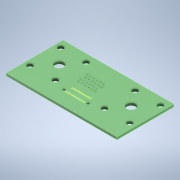
# Autodesk Inventor part: Cartridge PCB
Saved by Autodesk Inventor 2021 (Build 250183000, 183)
## iProperties
Created: 2020-04-22
Part Number: Cartridge PCB
Material: Generic
Document SubType Name: Modeling
Designer: jgray
Density: 1 g/cm^3
Appearance: Turquoise
Author: jgray
Autodesk Inventor part; units mm, degrees
ref_plane "YZ Plane" through (0, 0, 0) normal (1, 0, 0) x (0, 1, 0)
sketch "Sketch1" plane through (0, 0, 0) normal (0, 1, 0) x (-1, 0, 0)
  line L0 (-33.875, -17.375) -> (33.875, -17.375)
  line L1 (33.875, -17.375) -> (33.875, 17.375)
  line L2 (33.875, 17.375) -> (-33.875, 17.375)
  line L3 (-33.875, 17.375) -> (-33.875, -17.375)
  line L4 (-33.875, -17.375) -> (33.875, 17.375) construction
  line L5 (33.875, -17.375) -> (-33.875, 17.375) construction
  point P0 (0, 0)
  dimension "d0" = 67.75
  dimension "d1" = 34.75
  constraints: 12 end point, 2 midpoint, 2 parallel, 1 horizontal, 1 perpendicular
  measures "d0" distance of L2.end L1.end
  measures "d1" distance of L1.end L0.end
extrude "Extrusion1" add sketch "Sketch1" along normal blind 1.6
sketch "Sketch2" plane through (0, 1.6, 0) normal (0, 1, 0) x (1, 0, 0)
  line L0 (-33.875, 17.375) -> (-33.875, -17.375) projected
  line L1 (-33.875, -17.375) -> (33.875, -17.375) projected
  line L2 (33.875, -17.375) -> (33.875, 17.375) projected
  line L3 (33.875, 17.375) -> (-33.875, 17.375) projected
  line L4 (-35.405, 0) -> (38.2243, 0) construction
  line L5 (0, -28.3736) -> (0, 32.8828) construction
  line L6 (-37.7376, 3.2) -> (36.5002, 3.2) construction
  line L7 (22, -26.6494) -> (22, 29.2318) construction
  line L8 (-22, -24.9253) -> (-22, 32.8828) construction
  point P0 (0, 0)
  point P1 (-22, 3.2)
  point P2 (22, 3.2)
  dimension "d4" = 3.2
  dimension "d5" = 22
  dimension "d6" = 44
  constraints: 10 end point, 6 point on line, 3 vertical, 2 horizontal
  measures "d4" distance between parallel lines of L6 L4
  measures "d5" distance between parallel lines of L8 L5
  measures "d6" distance between parallel lines of L8 L7
hole "Hole1" at (-22, 1.6, -3.2) at (22, 1.6, -3.2) direction (0, -1, 0) diameter 5.5 end through all clearance for "Socket Head Cap Screw ISO 4762" size "M5" standard "ISO"
ref_plane "Work Plane1" through (0, 0, 17.375) normal (1, 0, 0) x (0, 0, -1)
ref_plane "Work Plane2" through (33.875, 0, 0) normal (0, 0, -1) x (-1, 0, 0)
sketch "Sketch3" plane through (0, 1.6, 0) normal (0, 1, 0) x (1, 0, 0)
  circle A0 centre (-22, 3.2) radius 2.75 projected
  circle A1 centre (22, 3.2) radius 2.75 projected
  line L0 (-33.875, 17.375) -> (-33.875, -17.375) projected
  line L1 (-33.875, -17.375) -> (33.875, -17.375) projected
  line L2 (33.875, -17.375) -> (33.875, 17.375) projected
  line L3 (33.875, 17.375) -> (-33.875, 17.375) projected
  line L4 (-39.0266, 3.2) -> (37.53, 3.2) construction
  line L5 (-15.4073, 6.3) -> (-2.3409, 6.3) construction
  line L6 (0, 20.8425) -> (0, -19.5249) construction
  line L7 (-36.2349, 0) -> (35.1135, 0) construction
  line L8 (-14.4073, 4.3) -> (-1.3409, 4.3) construction
  line L9 (-15.4073, 2.1) -> (-2.3409, 2.1) construction
  line L10 (-14.4073, 0.1) -> (-1.3409, 0.1) construction
  point P0 (0, 0)
  point P1 (-8, 6.3)
  point P2 (-6, 6.3)
  point P3 (-4, 6.3)
  point P4 (-2, 6.3)
  point P5 (0, 6.3)
  point P6 (2, 6.3)
  point P7 (-7, 4.3)
  point P8 (-5, 4.3)
  point P9 (-3, 4.3)
  point P10 (-1, 4.3)
  point P11 (1, 4.3)
  point P12 (3, 4.3)
  point P13 (-8, 2.1)
  point P14 (-6, 2.1)
  point P15 (-4, 2.1)
  point P16 (-2, 2.1)
  point P17 (0, 2.1)
  point P18 (2, 2.1)
  point P19 (-7, 0.1)
  point P20 (-5, 0.1)
  point P21 (-3, 0.1)
  point P22 (-1, 0.1)
  point P23 (1, 0.1)
  point P24 (3, 0.1)
  dimension "d16" = 2
  dimension "d25" = 2
  dimension "d35" = 2
  dimension "d49" = 2
  dimension "d51" = 1
  dimension "d52" = 2
  dimension "d53" = 1
  dimension "d54" = 2
  dimension "d55" = 2
  dimension "d56" = 2.2
  dimension "d57" = 8
  dimension "d111" = 1.1
  constraints: 14 end point, 9 horizontal, 7 point on line, 1 perpendicular, 1 vertical, 21 other
  measures "d16" distance of point (-8, 6.3) point (-6, 6.3)
  measures "d25" distance of point (-7, 4.3) point (-5, 4.3)
  measures "d35" distance of point (-8, 2.1) point (-6, 2.1)
  measures "d49" distance of point (-7, 0.1) point (-5, 0.1)
  measures "d51" horizontal distance of point (2, 6.3) point (3, 4.3)
  measures "d52" horizontal distance of point (-6, 6.3) point (-8, 2.1)
  measures "d53" horizontal distance of point (3, 0.1) point (2, 2.1)
  measures "d54" distance between parallel lines of L8 L5
  measures "d55" distance between parallel lines of L10 L9
  measures "d56" vertical distance of point (2, 2.1) point (3, 4.3)
  measures "d57" distance from line of point (-8, 6.3) L6
  measures "d111" distance from line of point (1, 4.3) L4
hole "Hole2" at (-8, 1.6, -6.3) at (-6, 1.6, -6.3) at (-4, 1.6, -6.3) at (-2, 1.6, -6.3) at (0, 1.6, -6.3) at (2, 1.6, -6.3) at (3, 1.6, -4.3) at (1, 1.6, -4.3) at (-1, 1.6, -4.3) at (-3, 1.6, -4.3) at (-5, 1.6, -4.3) at (-7, 1.6, -4.3) at (2, 1.6, -2.1) at (0, 1.6, -2.1) at (-2, 1.6, -2.1) at (-4, 1.6, -2.1) at (-6, 1.6, -2.1) at (-8, 1.6, -2.1) at (3, 1.6, -0.1) at (1, 1.6, -0.1) at (-1, 1.6, -0.1) at (-3, 1.6, -0.1) at (-5, 1.6, -0.1) at (-7, 1.6, -0.1) direction (0, -1, 0) diameter 0.8 end through all
sketch "Sketch4" plane through (0, 1.6, 0) normal (0, 1, 0) x (1, 0, 0)
  line L0 (0, 23.9201) -> (0, -23.9201) construction
  line L1 (-40.4387, 0) -> (47.2346, 0) construction
  line L2 (-12.2121, -8.55) -> (19.9504, -8.55) construction
  line L3 (-12.6831, -7.05) -> (19.9504, -7.05) construction
  line L4 (-42.6463, 3.2) -> (39.0543, 3.2) construction
  circle A0 centre (-5, 0.1) radius 0.4 construction
  circle A1 centre (-1, 0.1) radius 0.4 construction
  circle A2 centre (3, 0.1) radius 0.4 construction
  circle A3 centre (-6, 2.1) radius 0.4 construction
  circle A4 centre (-2, 2.1) radius 0.4 construction
  circle A5 centre (2, 2.1) radius 0.4 construction
  circle A6 centre (-5, 4.3) radius 0.4 construction
  circle A7 centre (-1, 4.3) radius 0.4 construction
  circle A8 centre (3, 4.3) radius 0.4 construction
  circle A9 centre (0, 6.3) radius 0.4 construction
  circle A10 centre (-4, 6.3) radius 0.4 construction
  circle A11 centre (-8, 6.3) radius 0.4 construction
  circle A12 centre (-6, 6.3) radius 0.4 construction
  circle A13 centre (-2, 6.3) radius 0.4 construction
  circle A14 centre (2, 6.3) radius 0.4 construction
  circle A15 centre (1, 4.3) radius 0.4 construction
  circle A16 centre (-3, 4.3) radius 0.4 construction
  circle A17 centre (-7, 4.3) radius 0.4 construction
  circle A18 centre (0, 2.1) radius 0.4 construction
  circle A19 centre (-4, 2.1) radius 0.4 construction
  circle A20 centre (-8, 2.1) radius 0.4 construction
  circle A21 centre (1, 0.1) radius 0.4 construction
  circle A22 centre (-3, 0.1) radius 0.4 construction
  circle A23 centre (-7, 0.1) radius 0.4 construction
  circle A24 centre (-22, 3.2) radius 2.75 construction
  circle A25 centre (22, 3.2) radius 2.75 construction
  line L5 (-33.875, 17.375) -> (-33.875, -17.375) construction
  line L6 (-33.875, -17.375) -> (33.875, -17.375) construction
  line L7 (33.875, -17.375) -> (33.875, 17.375) construction
  line L8 (33.875, 17.375) -> (-33.875, 17.375) construction
  point P0 (0, 0)
  point P1 (0, 0)
  point P2 (-7.4, -8.55)
  point P3 (7.4, -8.55)
  dimension "d65" = 1.5
  dimension "d66" = 14.8
  dimension "d67" = 10.25
  constraints: 10 end point, 6 point on line, 4 horizontal, 2 midpoint, 1 symmetric about line, 1 vertical
  measures "d65" distance between parallel lines of L3 L2
  measures "d66" distance of point (7.4, -8.55) point (-7.4, -8.55)
  measures "d67" distance between parallel lines of L4 L3
hole "Hole3" at (-7.4, 1.6, 8.55) at (7.4, 1.6, 8.55) direction (0, -1, 0) diameter 1.45 end through all
sketch "Sketch5" plane through (0, 1.6, 0) normal (0, 1, 0) x (1, 0, 0)
  line L0 (-11.5772, -5.15) -> (25.3732, -5.15) construction
  line L1 (-5.35, -5.7) -> (-5.85, -5.7)
  line L2 (-5.85, -5.7) -> (-5.85, -4.6)
  line L3 (-5.85, -4.6) -> (-5.35, -4.6)
  line L4 (-5.35, -4.6) -> (-5.35, -5.7)
  line L5 (-5.35, -5.7) -> (-5.85, -4.6) construction
  line L6 (-5.85, -5.7) -> (-5.35, -4.6) construction
  line L7 (0, 27.1403) -> (0, -35.4956) construction
  line L8 (-12.2121, -8.55) -> (19.9504, -8.55) construction
  line L9 (-12.6831, -7.05) -> (19.9504, -7.05) construction
  circle A0 centre (-7.4, -8.55) radius 0.725 construction
  circle A1 centre (7.4, -8.55) radius 0.725 construction
  circle A2 centre (-5, 0.1) radius 0.4 construction
  circle A3 centre (-1, 0.1) radius 0.4 construction
  circle A4 centre (3, 0.1) radius 0.4 construction
  circle A5 centre (-6, 2.1) radius 0.4 construction
  circle A6 centre (-2, 2.1) radius 0.4 construction
  circle A7 centre (2, 2.1) radius 0.4 construction
  circle A8 centre (-5, 4.3) radius 0.4 construction
  circle A9 centre (-1, 4.3) radius 0.4 construction
  circle A10 centre (3, 4.3) radius 0.4 construction
  circle A11 centre (0, 6.3) radius 0.4 construction
  circle A12 centre (-4, 6.3) radius 0.4 construction
  circle A13 centre (-8, 6.3) radius 0.4 construction
  circle A14 centre (-6, 6.3) radius 0.4 construction
  circle A15 centre (-2, 6.3) radius 0.4 construction
  circle A16 centre (2, 6.3) radius 0.4 construction
  circle A17 centre (1, 4.3) radius 0.4 construction
  circle A18 centre (-3, 4.3) radius 0.4 construction
  circle A19 centre (-7, 4.3) radius 0.4 construction
  circle A20 centre (0, 2.1) radius 0.4 construction
  circle A21 centre (-4, 2.1) radius 0.4 construction
  circle A22 centre (-8, 2.1) radius 0.4 construction
  circle A23 centre (1, 0.1) radius 0.4 construction
  circle A24 centre (-3, 0.1) radius 0.4 construction
  circle A25 centre (-7, 0.1) radius 0.4 construction
  circle A26 centre (-22, 3.2) radius 2.75 construction
  circle A27 centre (22, 3.2) radius 2.75 construction
  line L10 (-33.875, 17.375) -> (-33.875, -17.375) construction
  line L11 (-33.875, -17.375) -> (33.875, -17.375) construction
  line L12 (33.875, -17.375) -> (33.875, 17.375) construction
  line L13 (33.875, 17.375) -> (-33.875, 17.375) construction
  line L14 (-5.05, -5.7) -> (-5.05, -4.6)
  line L15 (-5.05, -4.6) -> (-4.55, -4.6)
  line L16 (-4.55, -5.7) -> (-5.05, -4.6) construction
  line L17 (-5.05, -5.7) -> (-4.55, -4.6) construction
  line L18 (-4.55, -4.6) -> (-4.55, -5.7)
  line L19 (-4.55, -5.7) -> (-5.05, -5.7)
  line L20 (-4.25, -5.7) -> (-4.25, -4.6)
  line L21 (-4.25, -4.6) -> (-3.75, -4.6)
  line L22 (-3.75, -5.7) -> (-4.25, -4.6) construction
  line L23 (-4.25, -5.7) -> (-3.75, -4.6) construction
  line L24 (-3.75, -4.6) -> (-3.75, -5.7)
  line L25 (-3.75, -5.7) -> (-4.25, -5.7)
  line L26 (-3.45, -5.7) -> (-3.45, -4.6)
  line L27 (-3.45, -4.6) -> (-2.95, -4.6)
  line L28 (-2.95, -5.7) -> (-3.45, -4.6) construction
  line L29 (-3.45, -5.7) -> (-2.95, -4.6) construction
  line L30 (-2.95, -4.6) -> (-2.95, -5.7)
  line L31 (-2.95, -5.7) -> (-3.45, -5.7)
  line L32 (-2.65, -5.7) -> (-2.65, -4.6)
  line L33 (-2.65, -4.6) -> (-2.15, -4.6)
  line L34 (-2.15, -5.7) -> (-2.65, -4.6) construction
  line L35 (-2.65, -5.7) -> (-2.15, -4.6) construction
  line L36 (-2.15, -4.6) -> (-2.15, -5.7)
  line L37 (-2.15, -5.7) -> (-2.65, -5.7)
  line L38 (-1.85, -5.7) -> (-1.85, -4.6)
  line L39 (-1.85, -4.6) -> (-1.35, -4.6)
  line L40 (-1.35, -5.7) -> (-1.85, -4.6) construction
  line L41 (-1.85, -5.7) -> (-1.35, -4.6) construction
  line L42 (-1.35, -4.6) -> (-1.35, -5.7)
  line L43 (-1.35, -5.7) -> (-1.85, -5.7)
  line L44 (-1.05, -5.7) -> (-1.05, -4.6)
  line L45 (-1.05, -4.6) -> (-0.55, -4.6)
  line L46 (-0.55, -5.7) -> (-1.05, -4.6) construction
  line L47 (-1.05, -5.7) -> (-0.55, -4.6) construction
  line L48 (-0.55, -4.6) -> (-0.55, -5.7)
  line L49 (-0.55, -5.7) -> (-1.05, -5.7)
  line L50 (-0.25, -5.7) -> (-0.25, -4.6)
  line L51 (-0.25, -4.6) -> (0.25, -4.6)
  line L52 (0.25, -5.7) -> (-0.25, -4.6) construction
  line L53 (-0.25, -5.7) -> (0.25, -4.6) construction
  line L54 (0.25, -4.6) -> (0.25, -5.7)
  line L55 (0.25, -5.7) -> (-0.25, -5.7)
  line L56 (0.55, -5.7) -> (0.55, -4.6)
  line L57 (0.55, -4.6) -> (1.05, -4.6)
  line L58 (1.05, -5.7) -> (0.55, -4.6) construction
  line L59 (0.55, -5.7) -> (1.05, -4.6) construction
  line L60 (1.05, -4.6) -> (1.05, -5.7)
  line L61 (1.05, -5.7) -> (0.55, -5.7)
  line L62 (1.35, -5.7) -> (1.35, -4.6)
  line L63 (1.35, -4.6) -> (1.85, -4.6)
  line L64 (1.85, -5.7) -> (1.35, -4.6) construction
  line L65 (1.35, -5.7) -> (1.85, -4.6) construction
  line L66 (1.85, -4.6) -> (1.85, -5.7)
  line L67 (1.85, -5.7) -> (1.35, -5.7)
  line L68 (2.15, -5.7) -> (2.15, -4.6)
  line L69 (2.15, -4.6) -> (2.65, -4.6)
  line L70 (2.65, -5.7) -> (2.15, -4.6) construction
  line L71 (2.15, -5.7) -> (2.65, -4.6) construction
  line L72 (2.65, -4.6) -> (2.65, -5.7)
  line L73 (2.65, -5.7) -> (2.15, -5.7)
  line L74 (2.95, -5.7) -> (2.95, -4.6)
  line L75 (2.95, -4.6) -> (3.45, -4.6)
  line L76 (3.45, -5.7) -> (2.95, -4.6) construction
  line L77 (2.95, -5.7) -> (3.45, -4.6) construction
  line L78 (3.45, -4.6) -> (3.45, -5.7)
  line L79 (3.45, -5.7) -> (2.95, -5.7)
  line L80 (3.75, -5.7) -> (3.75, -4.6)
  line L81 (3.75, -4.6) -> (4.25, -4.6)
  line L82 (4.25, -5.7) -> (3.75, -4.6) construction
  line L83 (3.75, -5.7) -> (4.25, -4.6) construction
  line L84 (4.25, -4.6) -> (4.25, -5.7)
  line L85 (4.25, -5.7) -> (3.75, -5.7)
  line L86 (4.55, -5.7) -> (4.55, -4.6)
  line L87 (4.55, -4.6) -> (5.05, -4.6)
  line L88 (5.05, -5.7) -> (4.55, -4.6) construction
  line L89 (4.55, -5.7) -> (5.05, -4.6) construction
  line L90 (5.05, -4.6) -> (5.05, -5.7)
  line L91 (5.05, -5.7) -> (4.55, -5.7)
  line L92 (5.35, -5.7) -> (5.35, -4.6)
  line L93 (5.35, -4.6) -> (5.85, -4.6)
  line L94 (5.85, -5.7) -> (5.35, -4.6) construction
  line L95 (5.35, -5.7) -> (5.85, -4.6) construction
  line L96 (5.85, -4.6) -> (5.85, -5.7)
  line L97 (5.85, -5.7) -> (5.35, -5.7)
  line L98 (-5.85, -9.5) -> (-5.85, -8.4)
  line L99 (-5.85, -8.4) -> (-5.35, -8.4)
  line L100 (-5.35, -9.5) -> (-5.85, -8.4) construction
  line L101 (-5.85, -9.5) -> (-5.35, -8.4) construction
  line L102 (-5.35, -8.4) -> (-5.35, -9.5)
  line L103 (-5.35, -9.5) -> (-5.85, -9.5)
  line L104 (-5.05, -9.5) -> (-5.05, -8.4)
  line L105 (-5.05, -8.4) -> (-4.55, -8.4)
  line L106 (-4.55, -9.5) -> (-5.05, -8.4) construction
  line L107 (-5.05, -9.5) -> (-4.55, -8.4) construction
  line L108 (-4.55, -8.4) -> (-4.55, -9.5)
  line L109 (-4.55, -9.5) -> (-5.05, -9.5)
  line L110 (-4.25, -9.5) -> (-4.25, -8.4)
  line L111 (-4.25, -8.4) -> (-3.75, -8.4)
  line L112 (-3.75, -9.5) -> (-4.25, -8.4) construction
  line L113 (-4.25, -9.5) -> (-3.75, -8.4) construction
  line L114 (-3.75, -8.4) -> (-3.75, -9.5)
  line L115 (-3.75, -9.5) -> (-4.25, -9.5)
  line L116 (-3.45, -9.5) -> (-3.45, -8.4)
  line L117 (-3.45, -8.4) -> (-2.95, -8.4)
  line L118 (-2.95, -9.5) -> (-3.45, -8.4) construction
  line L119 (-3.45, -9.5) -> (-2.95, -8.4) construction
  line L120 (-2.95, -8.4) -> (-2.95, -9.5)
  line L121 (-2.95, -9.5) -> (-3.45, -9.5)
  line L122 (-2.65, -9.5) -> (-2.65, -8.4)
  line L123 (-2.65, -8.4) -> (-2.15, -8.4)
  line L124 (-2.15, -9.5) -> (-2.65, -8.4) construction
  line L125 (-2.65, -9.5) -> (-2.15, -8.4) construction
  line L126 (-2.15, -8.4) -> (-2.15, -9.5)
  line L127 (-2.15, -9.5) -> (-2.65, -9.5)
  line L128 (-1.85, -9.5) -> (-1.85, -8.4)
  line L129 (-1.85, -8.4) -> (-1.35, -8.4)
  line L130 (-1.35, -9.5) -> (-1.85, -8.4) construction
  line L131 (-1.85, -9.5) -> (-1.35, -8.4) construction
  line L132 (-1.35, -8.4) -> (-1.35, -9.5)
  line L133 (-1.35, -9.5) -> (-1.85, -9.5)
  line L134 (-1.05, -9.5) -> (-1.05, -8.4)
  line L135 (-1.05, -8.4) -> (-0.55, -8.4)
  line L136 (-0.55, -9.5) -> (-1.05, -8.4) construction
  line L137 (-1.05, -9.5) -> (-0.55, -8.4) construction
  line L138 (-0.55, -8.4) -> (-0.55, -9.5)
  line L139 (-0.55, -9.5) -> (-1.05, -9.5)
  line L140 (-0.25, -9.5) -> (-0.25, -8.4)
  line L141 (-0.25, -8.4) -> (0.25, -8.4)
  line L142 (0.25, -9.5) -> (-0.25, -8.4) construction
  line L143 (-0.25, -9.5) -> (0.25, -8.4) construction
  line L144 (0.25, -8.4) -> (0.25, -9.5)
  line L145 (0.25, -9.5) -> (-0.25, -9.5)
  line L146 (0.55, -9.5) -> (0.55, -8.4)
  line L147 (0.55, -8.4) -> (1.05, -8.4)
  line L148 (1.05, -9.5) -> (0.55, -8.4) construction
  line L149 (0.55, -9.5) -> (1.05, -8.4) construction
  line L150 (1.05, -8.4) -> (1.05, -9.5)
  line L151 (1.05, -9.5) -> (0.55, -9.5)
  line L152 (1.35, -9.5) -> (1.35, -8.4)
  line L153 (1.35, -8.4) -> (1.85, -8.4)
  line L154 (1.85, -9.5) -> (1.35, -8.4) construction
  line L155 (1.35, -9.5) -> (1.85, -8.4) construction
  line L156 (1.85, -8.4) -> (1.85, -9.5)
  line L157 (1.85, -9.5) -> (1.35, -9.5)
  line L158 (2.15, -9.5) -> (2.15, -8.4)
  line L159 (2.15, -8.4) -> (2.65, -8.4)
  line L160 (2.65, -9.5) -> (2.15, -8.4) construction
  line L161 (2.15, -9.5) -> (2.65, -8.4) construction
  line L162 (2.65, -8.4) -> (2.65, -9.5)
  line L163 (2.65, -9.5) -> (2.15, -9.5)
  line L164 (2.95, -9.5) -> (2.95, -8.4)
  line L165 (2.95, -8.4) -> (3.45, -8.4)
  line L166 (3.45, -9.5) -> (2.95, -8.4) construction
  line L167 (2.95, -9.5) -> (3.45, -8.4) construction
  line L168 (3.45, -8.4) -> (3.45, -9.5)
  line L169 (3.45, -9.5) -> (2.95, -9.5)
  line L170 (3.75, -9.5) -> (3.75, -8.4)
  line L171 (3.75, -8.4) -> (4.25, -8.4)
  line L172 (4.25, -9.5) -> (3.75, -8.4) construction
  line L173 (3.75, -9.5) -> (4.25, -8.4) construction
  line L174 (4.25, -8.4) -> (4.25, -9.5)
  line L175 (4.25, -9.5) -> (3.75, -9.5)
  line L176 (4.55, -9.5) -> (4.55, -8.4)
  line L177 (4.55, -8.4) -> (5.05, -8.4)
  line L178 (5.05, -9.5) -> (4.55, -8.4) construction
  line L179 (4.55, -9.5) -> (5.05, -8.4) construction
  line L180 (5.05, -8.4) -> (5.05, -9.5)
  line L181 (5.05, -9.5) -> (4.55, -9.5)
  line L182 (5.35, -9.5) -> (5.35, -8.4)
  line L183 (5.35, -8.4) -> (5.85, -8.4)
  line L184 (5.85, -9.5) -> (5.35, -8.4) construction
  line L185 (5.35, -9.5) -> (5.85, -8.4) construction
  line L186 (5.85, -8.4) -> (5.85, -9.5)
  line L187 (5.85, -9.5) -> (5.35, -9.5)
  point P0 (0, 0)
  point P1 (-5.6, -5.15)
  point P2 (-4.8, -5.15)
  point P3 (-4, -5.15)
  point P4 (-3.2, -5.15)
  point P5 (-2.4, -5.15)
  point P6 (-1.6, -5.15)
  point P7 (-0.8, -5.15)
  point P8 (0, -5.15)
  point P9 (0.8, -5.15)
  point P10 (1.6, -5.15)
  point P11 (2.4, -5.15)
  point P12 (3.2, -5.15)
  point P13 (4, -5.15)
  point P14 (4.8, -5.15)
  point P15 (5.6, -5.15)
  point P16 (-5.6, -8.95)
  point P17 (-4.8, -8.95)
  point P18 (-4, -8.95)
  point P19 (-3.2, -8.95)
  point P20 (-2.4, -8.95)
  point P21 (-1.6, -8.95)
  point P22 (-0.8, -8.95)
  point P23 (0, -8.95)
  point P24 (0.8, -8.95)
  point P25 (1.6, -8.95)
  point P26 (2.4, -8.95)
  point P27 (3.2, -8.95)
  point P28 (4, -8.95)
  point P29 (4.8, -8.95)
  point P30 (5.6, -8.95)
  dimension "d75" = 0.5
  dimension "d76" = 1.1
  dimension "d79" = 0.8
  dimension "d82" = 3.8
  constraints: 364 end point, 60 midpoint, 3 horizontal, 2 parallel, 2 point on line, 2 vertical, 1 perpendicular, 321 other
  measures "d75" distance of L2.end L3.end
  measures "d76" distance of L1.end L2.end
  measures "d79" distance of point (-5.6, -5.15) point (-4.8, -5.15)
  measures "d82" distance of point (-5.6, -5.15) point (-5.6, -8.95)
extrude "Extrusion2" add sketch "Sketch5" along normal blind 0.01
sketch "Sketch6" plane through (0, 1.6, 0) normal (0, 1, 0) x (1, 0, 0)
  line L0 (-22.6077, 5.5) -> (-19.9207, 5.5) construction
  circle A0 centre (22, 5.5) radius 6.35 construction
  circle A1 centre (-22, 3.2) radius 6.35 construction
  line L1 (34, 17.625) -> (34, -17.625) construction
  line L2 (-34, 17.625) -> (34, 17.625) construction
  line L3 (-34, -17.625) -> (-34, 17.625) construction
  line L4 (34, -17.625) -> (-34, -17.625) construction
  line L5 (9.1, -9.9) -> (9.1, -4.1) construction
  line L6 (-9.1, -9.9) -> (9.1, -9.9) construction
  line L7 (-9.1, -4.1) -> (-9.1, -9.9) construction
  line L8 (9.1, -4.1) -> (-9.1, -4.1) construction
  line L9 (30.5, 12.6) -> (30.5, -6.2) construction
  line L10 (30.5, -6.2) -> (-30.5, -6.2) construction
  line L11 (-30.5, -6.2) -> (-30.5, 12.6) construction
  line L12 (-30.5, 12.6) -> (30.5, 12.6) construction
  line L13 (30.5, 12.6) -> (-30.5, -6.2) construction
  line L14 (30.5, -6.2) -> (-30.5, 12.6) construction
  line L15 (-1.85, -9.5) -> (-1.85, -8.4) projected
  line L16 (-1.85, -8.4) -> (-1.35, -8.4) projected
  line L17 (-1.35, -8.4) -> (-1.35, -9.5) projected
  line L18 (-1.35, -9.5) -> (-1.85, -9.5) projected
  line L19 (5.85, -8.4) -> (5.85, -9.5) projected
  line L20 (5.85, -9.5) -> (5.35, -9.5) projected
  line L21 (5.35, -9.5) -> (5.35, -8.4) projected
  line L22 (5.35, -8.4) -> (5.85, -8.4) projected
  line L23 (4.25, -5.7) -> (3.75, -5.7) projected
  line L24 (3.75, -5.7) -> (3.75, -4.6) projected
  line L25 (3.75, -4.6) -> (4.25, -4.6) projected
  line L26 (4.25, -4.6) -> (4.25, -5.7) projected
  line L27 (3.75, -8.4) -> (4.25, -8.4) projected
  line L28 (4.25, -8.4) -> (4.25, -9.5) projected
  line L29 (4.25, -9.5) -> (3.75, -9.5) projected
  line L30 (3.75, -9.5) -> (3.75, -8.4) projected
  line L31 (-1.05, -8.4) -> (-0.55, -8.4) projected
  line L32 (-0.55, -8.4) -> (-0.55, -9.5) projected
  line L33 (-0.55, -9.5) -> (-1.05, -9.5) projected
  line L34 (-1.05, -9.5) -> (-1.05, -8.4) projected
  line L35 (-0.55, -5.7) -> (-1.05, -5.7) projected
  line L36 (-1.05, -5.7) -> (-1.05, -4.6) projected
  line L37 (-1.05, -4.6) -> (-0.55, -4.6) projected
  line L38 (-0.55, -4.6) -> (-0.55, -5.7) projected
  line L39 (-4.25, -9.5) -> (-4.25, -8.4) projected
  line L40 (-4.25, -8.4) -> (-3.75, -8.4) projected
  line L41 (-3.75, -8.4) -> (-3.75, -9.5) projected
  line L42 (-3.75, -9.5) -> (-4.25, -9.5) projected
  line L43 (-2.95, -9.5) -> (-3.45, -9.5) projected
  line L44 (-3.45, -9.5) -> (-3.45, -8.4) projected
  line L45 (-3.45, -8.4) -> (-2.95, -8.4) projected
  line L46 (-2.95, -8.4) -> (-2.95, -9.5) projected
  line L47 (-2.65, -8.4) -> (-2.15, -8.4) projected
  line L48 (-2.15, -8.4) -> (-2.15, -9.5) projected
  line L49 (-2.15, -9.5) -> (-2.65, -9.5) projected
  line L50 (-2.65, -9.5) -> (-2.65, -8.4) projected
  line L51 (5.05, -8.4) -> (5.05, -9.5) projected
  line L52 (5.05, -9.5) -> (4.55, -9.5) projected
  line L53 (4.55, -9.5) -> (4.55, -8.4) projected
  line L54 (4.55, -8.4) -> (5.05, -8.4) projected
  line L55 (0.55, -5.7) -> (0.55, -4.6) projected
  line L56 (0.55, -4.6) -> (1.05, -4.6) projected
  line L57 (1.05, -4.6) -> (1.05, -5.7) projected
  line L58 (1.05, -5.7) -> (0.55, -5.7) projected
  line L59 (-4.25, -5.7) -> (-4.25, -4.6) projected
  line L60 (-4.25, -4.6) -> (-3.75, -4.6) projected
  line L61 (-3.75, -4.6) -> (-3.75, -5.7) projected
  line L62 (-3.75, -5.7) -> (-4.25, -5.7) projected
  line L63 (3.45, -9.5) -> (2.95, -9.5) projected
  line L64 (2.95, -9.5) -> (2.95, -8.4) projected
  line L65 (2.95, -8.4) -> (3.45, -8.4) projected
  line L66 (3.45, -8.4) -> (3.45, -9.5) projected
  line L67 (1.85, -8.4) -> (1.85, -9.5) projected
  line L68 (1.85, -9.5) -> (1.35, -9.5) projected
  line L69 (1.35, -9.5) -> (1.35, -8.4) projected
  line L70 (1.35, -8.4) -> (1.85, -8.4) projected
  line L71 (-3.45, -4.6) -> (-2.95, -4.6) projected
  line L72 (-2.95, -4.6) -> (-2.95, -5.7) projected
  line L73 (-2.95, -5.7) -> (-3.45, -5.7) projected
  line L74 (-3.45, -5.7) -> (-3.45, -4.6) projected
  line L75 (1.35, -5.7) -> (1.35, -4.6) projected
  line L76 (1.35, -4.6) -> (1.85, -4.6) projected
  line L77 (1.85, -4.6) -> (1.85, -5.7) projected
  line L78 (1.85, -5.7) -> (1.35, -5.7) projected
  line L79 (5.35, -5.7) -> (5.35, -4.6) projected
  line L80 (5.35, -4.6) -> (5.85, -4.6) projected
  line L81 (5.85, -4.6) -> (5.85, -5.7) projected
  line L82 (5.85, -5.7) -> (5.35, -5.7) projected
  line L83 (0.55, -8.4) -> (1.05, -8.4) projected
  line L84 (1.05, -8.4) -> (1.05, -9.5) projected
  line L85 (1.05, -9.5) -> (0.55, -9.5) projected
  line L86 (0.55, -9.5) -> (0.55, -8.4) projected
  line L87 (2.15, -5.7) -> (2.15, -4.6) projected
  line L88 (2.15, -4.6) -> (2.65, -4.6) projected
  line L89 (2.65, -4.6) -> (2.65, -5.7) projected
  line L90 (2.65, -5.7) -> (2.15, -5.7) projected
  line L91 (-0.25, -5.7) -> (-0.25, -4.6) projected
  line L92 (-0.25, -4.6) -> (0.25, -4.6) projected
  line L93 (0.25, -4.6) -> (0.25, -5.7) projected
  line L94 (0.25, -5.7) -> (-0.25, -5.7) projected
  line L95 (-0.25, -9.5) -> (-0.25, -8.4) projected
  line L96 (-0.25, -8.4) -> (0.25, -8.4) projected
  line L97 (0.25, -8.4) -> (0.25, -9.5) projected
  line L98 (0.25, -9.5) -> (-0.25, -9.5) projected
  line L99 (-5.05, -9.5) -> (-5.05, -8.4) projected
  line L100 (-5.05, -8.4) -> (-4.55, -8.4) projected
  line L101 (-4.55, -8.4) -> (-4.55, -9.5) projected
  line L102 (-4.55, -9.5) -> (-5.05, -9.5) projected
  line L103 (-5.35, -9.5) -> (-5.85, -9.5) projected
  line L104 (-5.85, -9.5) -> (-5.85, -8.4) projected
  line L105 (-5.85, -8.4) -> (-5.35, -8.4) projected
  line L106 (-5.35, -8.4) -> (-5.35, -9.5) projected
  line L107 (-5.85, -4.6) -> (-5.35, -4.6) projected
  line L108 (-5.35, -4.6) -> (-5.35, -5.7) projected
  line L109 (-5.35, -5.7) -> (-5.85, -5.7) projected
  line L110 (-5.85, -5.7) -> (-5.85, -4.6) projected
  line L111 (-4.55, -5.7) -> (-5.05, -5.7) projected
  line L112 (-5.05, -5.7) -> (-5.05, -4.6) projected
  line L113 (-5.05, -4.6) -> (-4.55, -4.6) projected
  line L114 (-4.55, -4.6) -> (-4.55, -5.7) projected
  line L115 (2.65, -9.5) -> (2.15, -9.5) projected
  line L116 (2.15, -9.5) -> (2.15, -8.4) projected
  line L117 (2.15, -8.4) -> (2.65, -8.4) projected
  line L118 (2.65, -8.4) -> (2.65, -9.5) projected
  line L119 (3.45, -5.7) -> (2.95, -5.7) projected
  line L120 (2.95, -5.7) -> (2.95, -4.6) projected
  line L121 (2.95, -4.6) -> (3.45, -4.6) projected
  line L122 (3.45, -4.6) -> (3.45, -5.7) projected
  line L123 (5.05, -5.7) -> (4.55, -5.7) projected
  line L124 (4.55, -5.7) -> (4.55, -4.6) projected
  line L125 (4.55, -4.6) -> (5.05, -4.6) projected
  line L126 (5.05, -4.6) -> (5.05, -5.7) projected
  line L127 (-1.35, -5.7) -> (-1.85, -5.7) projected
  line L128 (-1.85, -5.7) -> (-1.85, -4.6) projected
  line L129 (-1.85, -4.6) -> (-1.35, -4.6) projected
  line L130 (-1.35, -4.6) -> (-1.35, -5.7) projected
  line L131 (-2.65, -4.6) -> (-2.15, -4.6) projected
  line L132 (-2.15, -4.6) -> (-2.15, -5.7) projected
  line L133 (-2.15, -5.7) -> (-2.65, -5.7) projected
  line L134 (-2.65, -5.7) -> (-2.65, -4.6) projected
  circle A2 centre (-7.4, -8.55) radius 0.725 projected
  circle A3 centre (7.4, -8.55) radius 0.725 projected
  circle A4 centre (-5, 0.1) radius 0.4 projected
  circle A5 centre (-1, 0.1) radius 0.4 projected
  circle A6 centre (3, 0.1) radius 0.4 projected
  circle A7 centre (-6, 2.1) radius 0.4 projected
  circle A8 centre (-2, 2.1) radius 0.4 projected
  circle A9 centre (2, 2.1) radius 0.4 projected
  circle A10 centre (-5, 4.3) radius 0.4 projected
  circle A11 centre (-1, 4.3) radius 0.4 projected
  circle A12 centre (3, 4.3) radius 0.4 projected
  circle A13 centre (0, 6.3) radius 0.4 projected
  circle A14 centre (-4, 6.3) radius 0.4 projected
  circle A15 centre (-8, 6.3) radius 0.4 projected
  circle A16 centre (-6, 6.3) radius 0.4 projected
  circle A17 centre (-2, 6.3) radius 0.4 projected
  circle A18 centre (2, 6.3) radius 0.4 projected
  circle A19 centre (1, 4.3) radius 0.4 projected
  circle A20 centre (-3, 4.3) radius 0.4 projected
  circle A21 centre (-7, 4.3) radius 0.4 projected
  circle A22 centre (0, 2.1) radius 0.4 projected
  circle A23 centre (-4, 2.1) radius 0.4 projected
  circle A24 centre (-8, 2.1) radius 0.4 projected
  circle A25 centre (1, 0.1) radius 0.4 projected
  circle A26 centre (-3, 0.1) radius 0.4 projected
  circle A27 centre (-7, 0.1) radius 0.4 projected
  circle A28 centre (-22, 3.2) radius 2.75 projected
  circle A29 centre (22, 3.2) radius 2.75 projected
  line L135 (-33.875, 17.375) -> (-33.875, -17.375) projected
  line L136 (-33.875, -17.375) -> (33.875, -17.375) projected
  line L137 (33.875, -17.375) -> (33.875, 17.375) projected
  line L138 (33.875, 17.375) -> (-33.875, 17.375) projected
  line L139 (-39.3225, 3.2) -> (37.1971, 3.2) construction
  point P0 (0, 0)
  point P1 (34.125, -15.125)
  point P2 (0, -17.625)
  point P3 (0, 3.2)
  point P4 (15, 12.6)
  point P5 (-15, 12.6)
  point P6 (-15, -6.2)
  point P7 (15, -6.2)
  dimension "d87" = 18.8
  dimension "d88" = 61
  dimension "d89" = 30
  dimension "d90" = 30
  constraints: 32 end point, 5 coincident, 5 point on line, 3 midpoint, 2 centre point, 2 horizontal, 2 parallel, 1 perpendicular, 1 other
  measures "d87" distance between parallel lines of L12 L10
  measures "d88" distance between parallel lines of L9 L11
  measures "d89" distance of point (15, 12.6) point (-15, 12.6)
  measures "d90" distance of point (15, -6.2) point (-15, -6.2)
hole "Hole4" at (-15, 1.6, 6.2) at (15, 1.6, 6.2) at (15, 1.6, -12.6) at (-15, 1.6, -12.6) at (-30.5, 1.6, 6.2) at (-30.5, 1.6, -12.6) at (30.5, 1.6, -12.6) at (30.5, 1.6, 6.2) direction (0, -1, 0) diameter 3.4 end through all clearance for "Countersunk Flat Head Screw ISO 2009/7046" size "M3" standard "ISO"
sketch "Sketch7" plane through (0, 0, 0) normal (0, -1, 0) x (1, 0, 0)
  circle A0 centre (30.5, -12.6) radius 1.7 projected
  circle A1 centre (-30.5, 6.2) radius 1.7 projected
  circle A2 centre (15, -12.6) radius 1.7 projected
  circle A3 centre (-15, 6.2) radius 1.7 projected
  circle A4 centre (15, 6.2) radius 1.7 projected
  circle A5 centre (-15, -12.6) radius 1.7 projected
  circle A6 centre (-30.5, -12.6) radius 1.7 projected
  circle A7 centre (30.5, 6.2) radius 1.7 projected
  circle A8 centre (-7.4, 8.55) radius 0.725 projected
  circle A9 centre (7.4, 8.55) radius 0.725 projected
  circle A10 centre (-5, -0.1) radius 0.4 projected
  circle A11 centre (-1, -0.1) radius 0.4 projected
  circle A12 centre (3, -0.1) radius 0.4 projected
  circle A13 centre (-6, -2.1) radius 0.4 projected
  circle A14 centre (-2, -2.1) radius 0.4 projected
  circle A15 centre (2, -2.1) radius 0.4 projected
  circle A16 centre (-5, -4.3) radius 0.4 projected
  circle A17 centre (-1, -4.3) radius 0.4 projected
  circle A18 centre (3, -4.3) radius 0.4 projected
  circle A19 centre (0, -6.3) radius 0.4 projected
  circle A20 centre (-4, -6.3) radius 0.4 projected
  circle A21 centre (-8, -6.3) radius 0.4 projected
  circle A22 centre (-6, -6.3) radius 0.4 projected
  circle A23 centre (-2, -6.3) radius 0.4 projected
  circle A24 centre (2, -6.3) radius 0.4 projected
  circle A25 centre (1, -4.3) radius 0.4 projected
  circle A26 centre (-3, -4.3) radius 0.4 projected
  circle A27 centre (-7, -4.3) radius 0.4 projected
  circle A28 centre (0, -2.1) radius 0.4 projected
  circle A29 centre (-4, -2.1) radius 0.4 projected
  circle A30 centre (-8, -2.1) radius 0.4 projected
  circle A31 centre (1, -0.1) radius 0.4 projected
  circle A32 centre (-3, -0.1) radius 0.4 projected
  circle A33 centre (-7, -0.1) radius 0.4 projected
  circle A34 centre (-22, -3.2) radius 2.75 projected
  circle A35 centre (22, -3.2) radius 2.75 projected
  line L0 (-33.875, -17.375) -> (-33.875, 17.375) projected
  line L1 (33.875, -17.375) -> (-33.875, -17.375) projected
  line L2 (33.875, 17.375) -> (33.875, -17.375) projected
  line L3 (-33.875, 17.375) -> (33.875, 17.375) projected
  circle A36 centre (-22, -3.2) radius 5
  circle A37 centre (22, -3.2) radius 5
  line L4 (6.6, -7.3) -> (-11.6, -7.3)
  line L5 (-11.6, -7.3) -> (-11.6, 0.9)
  line L6 (-11.6, 0.9) -> (6.6, 0.9)
  line L7 (6.6, 0.9) -> (6.6, -7.3)
  line L8 (22, -3.2) -> (-22, -3.2)
  line L9 (-2.5, -13.1267) -> (-2.5, 10.1713)
  line L10 (17.6699, -5.7) -> (6.6, -5.7)
  line L11 (6.6, -5.7) -> (6.6, -0.7)
  line L12 (6.6, -0.7) -> (17.6699, -0.7)
  line L13 (-17.6699, -0.7) -> (-11.6, -0.7)
  line L14 (-11.6, -0.7) -> (-11.6, -5.7)
  line L15 (-11.6, -5.7) -> (-17.6699, -5.7)
  line L16 (-17.6699, -5.7) -> (-17.6699, -0.7)
  point P0 (0, 0)
  dimension "d98" = 10
  dimension "d99" = 10
  dimension "d100" = 18.2
  dimension "d101" = 8.2
  dimension "d102" = 10.4
  dimension "d103" = 19.5
  dimension "d104" = 5
  dimension "d110" = 5
  constraints: 26 end point, 5 parallel, 4 horizontal, 3 perpendicular, 2 coincident, 2 point on line, 1 vertical, 9 other
  measures "d100" distance of L5.end L6.end
  measures "d101" distance of L4.end L5.end
  measures "d102" distance from line of L8.end L5
  measures "d103" distance from line of A34.centre L9
  measures "d104" distance between parallel lines of L12 L10
  measures "d110" distance of L13.end L14.end
extrude "Extrusion3" add sketch "Sketch7" along normal blind 0.005 contours L8 L5 L15 A36 | A36 L13 L5 L8 | L8 L9 L4 L5 | L5 L6 L9 L8 | L9 L6 L7 L8 | L8 L7 L4 L9 | L8 A37 L10 L7 | L7 L12 A37 L8
sketch "Sketch8" plane through (0, 0, 0) normal (0, -1, 0) x (1, 0, 0)
  arc A0 (17.6699, -0.7) -> (17.6699, -5.7) centre (22, -3.2) ccw projected
  line L0 (17.6699, -5.7) -> (6.6, -5.7) projected
  line L1 (6.6, -5.7) -> (6.6, -7.3) projected
  line L2 (6.6, -7.3) -> (-11.6, -7.3) projected
  line L3 (-11.6, -7.3) -> (-11.6, -5.7) projected
  line L4 (-11.6, 0.9) -> (6.6, 0.9) projected
  line L5 (6.6, 0.9) -> (6.6, -0.7) projected
  line L6 (6.6, -0.7) -> (17.6699, -0.7) projected
  circle A1 centre (30.5, -12.6) radius 1.7 projected
  circle A2 centre (-30.5, 6.2) radius 1.7 projected
  circle A3 centre (15, -12.6) radius 1.7 projected
  circle A4 centre (-15, 6.2) radius 1.7 projected
  circle A5 centre (15, 6.2) radius 1.7 projected
  circle A6 centre (-15, -12.6) radius 1.7 projected
  circle A7 centre (-30.5, -12.6) radius 1.7 projected
  circle A8 centre (30.5, 6.2) radius 1.7 projected
  circle A9 centre (-7.4, 8.55) radius 0.725 projected
  circle A10 centre (7.4, 8.55) radius 0.725 projected
  circle A11 centre (-22, -3.2) radius 2.75 projected
  circle A12 centre (22, -3.2) radius 2.75 projected
  line L7 (-33.875, -17.375) -> (-33.875, 17.375) projected
  line L8 (33.875, -17.375) -> (-33.875, -17.375) projected
  line L9 (33.875, 17.375) -> (33.875, -17.375) projected
  line L10 (-33.875, 17.375) -> (33.875, 17.375) projected
  line L11 (-33.875, -17.375) -> (-33.875, 17.375) projected
  line L12 (33.875, 17.375) -> (33.875, -17.375) projected
  line L13 (-33.875, 17.375) -> (33.875, 17.375)
  line L14 (33.875, 17.375) -> (33.875, 11)
  line L15 (33.875, 11) -> (-33.875, 11)
  line L16 (-33.875, 11) -> (-33.875, 17.375)
  line L17 (-11.6, -5.7) -> (-17.6699, -5.7) projected
  arc A13 (-17.6699, -5.7) -> (-17.6699, -0.7) centre (-22, -3.2) ccw projected
  line L18 (-17.6699, -0.7) -> (-11.6, -0.7) projected
  line L19 (-11.6, -0.7) -> (-11.6, 0.9) projected
  point P0 (0, 0)
  dimension "d107" = 14.2
  constraints: 8 end point, 2 parallel, 2 point on line, 1 horizontal, 1 perpendicular
  measures "d107" distance from line of L15 A0.centre
extrude "Extrusion4" add sketch "Sketch8" along normal blind 0.005 contours L7 L10 L9 L15
body "Solid1"
